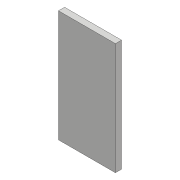
# Autodesk Inventor part: Buck_Bracket
Saved by Autodesk Inventor 2018 (Build 220112000, 112)
## iProperties
Created: 2019-11-08
Part Number: Buck_Bracket
Material: Generic
Document SubType Name: Modeling
Designer: Clevo
Density: 1 g/cm^3
Appearance: Default
Author: Clevo
Autodesk Inventor part; units mm, degrees
ref_plane "YZ Plane" through (0, 0, 0) normal (1, 0, 0) x (0, 1, 0)
ref_plane "XZ Plane" through (0, 0, 0) normal (0, 1, 0) x (-1, 0, 0)
ref_plane "XY Plane" through (0, 0, 0) normal (0, 0, 1) x (1, 0, 0)
sketch "Sketch1" plane through (0, 0, 0) normal (0, 1, 0) x (-1, 0, 0)
  line L0 (-14, -27.5) -> (14, -27.5)
  line L1 (14, -27.5) -> (14, 27.5)
  line L2 (14, 27.5) -> (-14, 27.5)
  line L3 (-14, 27.5) -> (-14, -27.5)
  line L4 (-14, -27.5) -> (14, 27.5) construction
  line L5 (14, -27.5) -> (-14, 27.5) construction
  point P0 (0, 0)
  dimension "d0" = 55
  dimension "d1" = 28
  constraints: 12 end point, 2 midpoint, 2 parallel, 1 horizontal, 1 perpendicular
  measures "d0" distance of L0.end L1.end
  measures "d1" distance of L0.start L0.end
extrude "Extrusion1" add sketch "Sketch1" along normal blind 3
sketch "Sketch2" plane through (0, 3, 0) normal (0, 1, 0) x (1, 0, 0)
  line L0 (10.75, 21.75) -> (-10.75, 21.75)
  line L1 (-10.75, 21.75) -> (-10.75, -21.75)
  line L2 (-10.75, -21.75) -> (10.75, -21.75)
  line L3 (10.75, -21.75) -> (10.75, 21.75)
  line L4 (10.75, 21.75) -> (-10.75, -21.75) construction
  line L5 (-10.75, 21.75) -> (10.75, -21.75) construction
  point P0 (0, 0)
  dimension "d4" = 43.5
  dimension "d5" = 21.5
  constraints: 12 end point, 2 midpoint, 2 parallel, 1 horizontal, 1 perpendicular
  measures "d4" distance of L0.end L1.end
  measures "d5" distance of L1.end L2.end
extrude "Extrusion2" cut sketch "Sketch2" against normal blind 1.6
body "Solid1"
